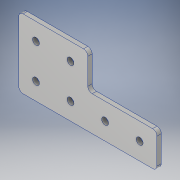
# Autodesk Inventor part: Sax Gusset
Saved by Autodesk Inventor 2018 (Build 220112000, 112)
## iProperties
Created: 2018-12-20
Part Number: Sax Gusset
Material: Aluminum 6061
Document SubType Name: Modeling
Designer: maste
Density: 2.7 g/cm^3
Appearance: Aluminum - Flat
Author: maste
Autodesk Inventor part; units mm, degrees
ref_plane "YZ Plane" through (0, 0, 0) normal (1, 0, 0) x (0, 1, 0)
ref_plane "XZ Plane" through (0, 0, 0) normal (0, 1, 0) x (-1, 0, 0)
ref_plane "XY Plane" through (0, 0, 0) normal (0, 0, 1) x (1, 0, 0)
sketch "Sketch1" plane through (0, 0, 0) normal (0, 0, 1) x (1, 0, 0)
  line L0 (0, 0) -> (0, 50.8)
  line L1 (0, 50.8) -> (50.8, 50.8)
  line L2 (50.8, 50.8) -> (50.8, 25.4)
  line L3 (50.8, 25.4) -> (101.6, 25.4)
  line L4 (101.6, 25.4) -> (101.6, 0)
  line L5 (101.6, 0) -> (0, 0)
  line L6 (0, 50.8) -> (12.7, 50.8) construction
  line L7 (12.7, 50.8) -> (12.7, 38.1) construction
  line L8 (12.7, 38.1) -> (38.1, 38.1) construction
  line L9 (38.1, 38.1) -> (38.1, 12.7) construction
  line L10 (38.1, 12.7) -> (12.7, 12.7) construction
  line L11 (12.7, 12.7) -> (63.5, 12.7) construction
  line L12 (63.5, 12.7) -> (88.9, 12.7) construction
  circle A0 centre (12.7, 38.1) radius 2.54
  circle A1 centre (38.1, 38.1) radius 2.54
  circle A2 centre (38.1, 12.7) radius 2.54
  circle A3 centre (12.7, 12.7) radius 2.54
  circle A4 centre (63.5, 12.7) radius 2.54
  circle A5 centre (88.9, 12.7) radius 2.54
  dimension "d0" = 50.8
  dimension "d1" = 50.8
  dimension "d2" = 25.4
  dimension "d3" = 50.8
  dimension "d4" = 12.7
  dimension "d5" = 12.7
  dimension "d6" = 25.4
  dimension "d8" = 25.4
  dimension "d9" = 25.4
  dimension "d10" = 50.8
  dimension "d11" = 25.4
  dimension "d12" = 5.08
  constraints: 26 end point, 8 perpendicular, 6 centre point, 6 coincident, 3 point on line, 2 vertical
  measures "d0" distance of L0.start L0.end
  measures "d1" distance of L0.end L1.end
  measures "d2" distance of L1.end L2.end
  measures "d3" distance of L2.end L3.end
  measures "d4" distance of L0.end L6.end
  measures "d5" distance of L6.end L7.end
  measures "d6" distance of L7.end L8.end
  measures "d8" distance of L8.end L9.end
  measures "d9" distance of L9.end L10.end
  measures "d10" distance of L10.end L11.end
  measures "d11" distance of L11.end L12.end
  measures "d12" diameter of A0
extrude "Extrusion1" add sketch "Sketch1" along normal blind 3.175
fillet "Fillet1" radius 3.175 6 edges at (50.8, 50.8, 1.5875) (50.8, 25.4, 1.5875) (0, 50.8, 1.5875) (0, 0, 1.5875) (101.6, 0, 1.5875) (101.6, 25.4, 1.5875)
body "Solid1"
